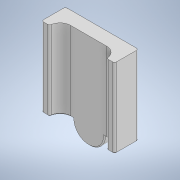
# Autodesk Inventor part: Test_SampleHolder_Plate_M8Screw_big
Saved by Autodesk Inventor 2021 (Build 250183000, 183)
## iProperties
Created: 2019-06-11
Part Number: Test_SampleHolder_Plate_M8Screw_big
Material: Generic
Document SubType Name: Modeling
Designer: Timo
Density: 1 g/cm^3
Appearance: Default
Author: Timo
Autodesk Inventor part; units mm, degrees
ref_plane "YZ Plane" through (0, 0, 0) normal (1, 0, 0) x (0, 1, 0)
ref_plane "XZ Plane" through (0, 0, 0) normal (0, 1, 0) x (-1, 0, 0)
ref_plane "XY Plane" through (0, 0, 0) normal (0, 0, 1) x (1, 0, 0)
sketch "Sketch1" plane through (0, 0, 0) normal (0, 0, 1) x (1, 0, 0)
  line L0 (-6.9, 7.5) -> (6.9, 7.5)
  line L1 (6.9, 7.5) -> (6.9, -7.5)
  line L2 (6.9, -7.5) -> (-6.9, -7.5)
  line L3 (-6.9, -7.5) -> (-6.9, 7.5)
  line L4 (0, -10.5) -> (0, 10.5) projected
  line L5 (-9.66, 0) -> (9.66, 0) projected
  point P0 (0, 0)
  dimension "d0" = 13.8
  dimension "d9" = 15
  constraints: 8 end point, 2 parallel, 1 horizontal, 1 perpendicular, 2 other
  measures "d0" distance of L0.start L0.end
  measures "d9" distance of L2.end L0.start
extrude "Extrusion1" add sketch "Sketch1" along normal blind 2.5
sketch "Sketch3" plane through (0, 0, 2.5) normal (0, 0, 1) x (1, 0, 0)
  line L0 (6.9, 7.5) -> (-6.9, 7.5) projected
  line L1 (-6.9, -7.5) -> (6.9, -7.5) projected
  line L2 (-6.9, 7.5) -> (-5.4, 7.5)
  line L3 (-5.4, 7.5) -> (-5.4, -7.5)
  line L4 (-5.4, -7.5) -> (-6.9, -7.5)
  line L5 (-6.9, -7.5) -> (-6.9, 7.5)
  line L6 (6.9, -7.5) -> (6.9, 7.5) projected
  line L7 (6.9, 7.5) -> (5.4, 7.5)
  line L8 (5.4, 7.5) -> (5.4, -7.5)
  line L9 (5.4, -7.5) -> (6.9, -7.5)
  line L10 (6.9, -7.5) -> (6.9, 7.5)
  point P0 (0, 0)
  point P1 (5.4, 7.5)
  point P2 (5.4, -7.5)
  dimension "d11" = 1.5
  dimension "d12" = 1.5
  constraints: 16 end point, 4 parallel, 2 horizontal, 2 perpendicular, 2 point on line
  measures "d11" distance between parallel lines of L6 L8
  measures "d12" distance between parallel lines of L5 L3
extrude "Extrusion3" add sketch "Sketch3" along normal blind 2 contours L6 L1 L8 L0 | L3 L1 L5 L0
fillet "Fillet2" radius 2 2 edges at (-5.4, 0, 2.5) (5.4, 0, 2.5)
fillet "Fillet2" radius 0.4 6 edges at (-5.4, 0, 4.5) (-6.9, 0, 4.5) (5.4, 0, 4.5) (6.9, 0, 4.5) (6.9, 0, 0) (-6.9, 0, 0)
sketch "Sketch4" plane through (0, 0, 2.5) normal (0, 0, 1) x (1, 0, 0)
  line L0 (-3.4, -7.5) -> (3.4, -7.5) projected
  arc A0 (-3, -7.5) -> (3, -7.5) centre (0, -7.5) ccw
  point P0 (0, 0)
  dimension "d17" = 3
  constraints: 2 point on circle, 1 centre point, 1 midpoint, 1 point on line
  measures "d17" radius of A0
extrude "Extrusion4" add sketch "Sketch4" against normal up to surface (2.5 mm away)
sketch "Sketch5" plane through (0, 0, 0) normal (0, 0, -1) x (-1, 0, 0)
  circle A0 centre (0, -0.5) radius 3.25
  line L0 (-3, -7.5) -> (-6.5, -7.5) construction
  line L1 (0, -15.3299) -> (0, 11.305) projected
  arc A1 (-3, -7.5) -> (3, -7.5) centre (0, -7.5) ccw projected
  point P0 (0, 0)
  dimension "d20" = 6.5
  dimension "d21" = 7
  constraints: 2 point on line, 1 centre point
  measures "d20" diameter of A0
  measures "d21" distance from line of L0 A0.centre
extrude "Extrusion5" cut sketch "Sketch5" against normal blind 1
chamfer "Chamfer2" distance 0.2 angle 45 16 edges at (0, -10.5, 2.5) (0, -10.5, 0) (-4.75, -7.5, 0) (6.7828, -7.5, 4.3828) (-6.7828, -7.5, 0.1172) (6.9, -7.5, 2.25) (6.1332, -7.5, 4.5) (-6.1332, -7.5, 4.5) (5.5082, -7.5, 4.4055) (-5.5082, -7.5, 4.4055) (-6.7828, -7.5, 4.3828) (4.6911, -7.5, 2.9725) (-4.6911, -7.5, 2.9725) (-3.2001, -7.5, 2.5) (3.2001, -7.5, 2.5) (-6.9, -7.5, 2.25)
chamfer "Chamfer3" distance 1 angle 30 1 edges at (3.25, -0.5, 0) measured on face at (-3.2395, -0.7615, 0.6667)
body "Solid1"
